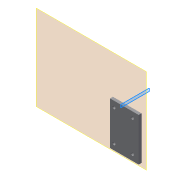
# Autodesk Inventor part: 03_Chipmount_v0
Saved by Autodesk Inventor 2019 (Build 230136000, 136)
## iProperties
Created: 2019-06-11
Part Number: 03_Chipmount_v0
Material: Generic
Document SubType Name: Modeling
Designer: diederichbenedict
Density: 1 g/cm^3
Appearance: Default
Author: diederichbenedict
Autodesk Inventor part; units mm, degrees
ref_plane "YZ Plane" through (0, 0, 0) normal (1, 0, 0) x (0, 1, 0)
ref_plane "XZ Plane" through (0, 0, 0) normal (0, 1, 0) x (-1, 0, 0)
ref_plane "XY Plane" through (0, 0, 0) normal (0, 0, 1) x (1, 0, 0)
ref_plane "Work Plane1" through (0, 0, 0) normal (0, 0, 1) x (1, 0, 0)
sketch "Sketch1" plane through (0, 0, 0) normal (0, 0, 1) x (1, 0, 0)
  circle A0 centre (-9.6869, -20.1071) radius 2.1 projected
  circle A1 centre (16.0451, 23.5027) radius 2.1 projected
  circle A2 centre (-9.6869, 23.5027) radius 2.1 projected
  circle A3 centre (16.0451, -20.1071) radius 2.1 projected
  line L0 (-36.7526, -23.851) -> (-36.7526, -20) projected
  line L1 (-36.7526, -20) -> (-105, -20) projected
  line L2 (-105, -20) -> (-105, 20) projected
  line L3 (-15, 20) -> (-105, 20) projected
  line L4 (-15, 20) -> (-15, -23.851) projected
  line L5 (-15, -23.851) -> (-36.7526, -23.851) projected
  circle A4 centre (-89.9475, 24.9475) radius 2.1 projected
  circle A5 centre (-39.9475, 24.9475) radius 2.1 projected
  circle A6 centre (-39.9475, 74.9475) radius 2.1 projected
  circle A7 centre (-89.9475, 74.9475) radius 2.1 projected
  circle A8 centre (-64.9475, 74.9475) radius 2.1 projected
  circle A9 centre (-39.9475, 49.9475) radius 2.1 projected
  circle A10 centre (-64.9475, 24.9475) radius 2.1 projected
  circle A11 centre (-89.9475, 49.9475) radius 2.1 projected
  line L6 (-115, 80) -> (25, 80) projected
  line L7 (-115, -28.406) -> (-115, 80) projected
  line L8 (25, -28.406) -> (-115, -28.406) projected
  line L9 (25, 80) -> (25, -28.406) projected
  line L10 (25, -28.406) -> (-15, -28.406)
  line L11 (-15, -28.406) -> (-15, 31.594)
  line L12 (-15, 31.594) -> (25, 31.594)
  line L13 (25, 31.594) -> (25, -28.406)
  point P0 (0, 0)
  dimension "d0" = 40
  dimension "d1" = 60
  constraints: 8 end point, 2 parallel, 1 horizontal, 1 perpendicular
  measures "d0" distance of L11.end L12.end
  measures "d1" distance of L10.end L11.end
extrude "Extrusion1" add sketch "Sketch1" along normal blind 4 contours L4 L11 L12 L9 L8
body "Solid1"
